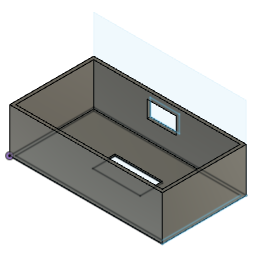
alarm_front v1 (Autodesk Fusion 360 design; units mm, degrees)
Autodesk Fusion 360 part; units mm, degrees
sketch "Sketch1" plane through (0, 0, 0) normal (0, 0, 1) x (1, 0, 0)
  line L0 (0, 0) -> (100, 0)
  line L1 (100, 0) -> (100, 55)
  line L2 (100, 55) -> (0, 55)
  line L3 (0, 55) -> (0, 0)
  line L4 (2, 2) -> (98, 2)
  line L5 (98, 2) -> (98, 53)
  line L6 (98, 53) -> (2, 53)
  line L7 (2, 53) -> (2, 2)
  line L8 (34.5, 34.5) -> (65.5, 34.5)
  line L9 (65.5, 34.5) -> (65.5, 20)
  line L10 (65.5, 20) -> (34.5, 20)
  line L11 (34.5, 20) -> (34.5, 34.5)
  dimension "d1" = -2
  dimension "d12" = 31
  dimension "d13" = 14.5
  dimension "d14" = 96
  dimension "d15" = 32.5
  dimension "d16" = 51
  dimension "d17" = 55
  dimension "d18" = 20
  constraint horizontal L0
  constraint vertical L1
  constraint horizontal L2
  constraint vertical L3
  constraint coincident L0.start L3.end
  constraint horizontal L8
  constraint vertical L9
  constraint horizontal L10
  constraint vertical L11
  measures "d12" distance of L8.start L8.end
  measures "d13" distance of L8 L10
  measures "d14" distance of L5 L7
  measures "d15" distance of L7 L11
  measures "d16" distance of L4 L6
  measures "d17" distance of L0 L2
  measures "d18" distance of L0 L10
extrude "Extrude1" add sketch "Sketch1" along normal blind 1 contours L4 L5 L6 L7
extrude "Extrude2" add sketch "Sketch1" along normal blind 4 contours L0 L1 L2 L3
extrude "Extrude3" add 1 faces at (34, 0.6667, 4) along direction (0, 0, 1) blind 50
sketch "Sketch2" plane through (0, 55, 0) normal (0, 1, 0) x (-1, 0, 0)
  line L0 (-100, 0) -> (0, 0)
  line L1 (0, 0) -> (0, 54)
  line L2 (0, 54) -> (-100, 54)
  line L3 (-100, 54) -> (-100, 0)
  line L4 (-56.0994, 24.0994) -> (-37.0994, 24.0994)
  line L5 (-37.0994, 24.0994) -> (-37.0994, 13.0994)
  line L6 (-37.0994, 13.0994) -> (-56.0994, 13.0994)
  line L7 (-56.0994, 13.0994) -> (-56.0994, 24.0994)
  dimension "d8" = 19
  dimension "d9" = 11
  constraint horizontal L4
  constraint vertical L5
  constraint horizontal L6
  constraint vertical L7
  measures "d8" distance of L4.start L4.end
  measures "d9" distance of L4.start L6.end
extrude "Extrude4" cut sketch "Sketch2" against normal blind 15 contours L4 L5 L6 L7
extrude "Extrude5" cut 1 faces at (34, 0.6667, 54) along direction (0, 0, -1) blind 25
